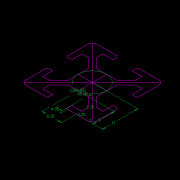
# Autodesk Inventor part: base2
Saved by Autodesk Inventor 2018 (Build 220112000, 112)
## iProperties
Created: 2022-02-17
Part Number: base2
Material: Generic
Document SubType Name: Modeling
Designer: kumpu
Density: 1 g/cm^3
Appearance: Default
Author: kumpu
Autodesk Inventor part; units mm, degrees
ref_plane "YZ Plane" through (0, 0, 0) normal (1, 0, 0) x (0, 1, 0)
ref_plane "XZ Plane" through (0, 0, 0) normal (0, 1, 0) x (-1, 0, 0)
ref_plane "XY Plane" through (0, 0, 0) normal (0, 0, 1) x (1, 0, 0)
sketch "Sketch1" plane through (0, 0, 0) normal (0, 1, 0) x (-1, 0, 0)
  line L0 (0, 0) -> (-14.4142, 14.4142)
  arc A0 (-13, 15) -> (-14.4142, 14.4142) centre (-13, 13) ccw
  line L1 (-13, 15) -> (-4.55, 15)
  line L2 (-4.55, 15) -> (-4, 14.45)
  line L3 (-4, 14.45) -> (-4, 12.75)
  line L4 (-4, 12.75) -> (-8.25, 12.75)
  line L5 (-8.25, 12.75) -> (-8.25, 10.0178)
  line L6 (-8.25, 10.0178) -> (-4.2322, 6)
  line L7 (-4.2322, 6) -> (0, 6)
  line L8 (0, 6) -> (0, 0)
  line L9 (0, 0) -> (14.4142, 14.4142)
  arc A1 (14.4142, 14.4142) -> (13, 15) centre (13, 13) ccw
  line L10 (13, 15) -> (4.55, 15)
  line L11 (4.55, 15) -> (4, 14.45)
  line L12 (4, 14.45) -> (4, 12.75)
  line L13 (4, 12.75) -> (8.25, 12.75)
  line L14 (8.25, 12.75) -> (8.25, 10.0178)
  line L15 (8.25, 10.0178) -> (4.2322, 6)
  line L16 (4.2322, 6) -> (0, 6)
  line L17 (-14.45, 4) -> (-12.75, 4)
  line L18 (-15, 4.55) -> (-14.45, 4)
  line L19 (-6, 4.2322) -> (-6, 0)
  line L20 (-6, 0) -> (0, 0)
  line L21 (-12.75, 4) -> (-12.75, 8.25)
  line L22 (-12.75, 8.25) -> (-10.0178, 8.25)
  line L23 (-10.0178, 8.25) -> (-6, 4.2322)
  line L24 (-15, 13) -> (-15, 4.55)
  arc A2 (-14.4142, 14.4142) -> (-15, 13) centre (-13, 13) ccw
  line L25 (0, 0) -> (-14.4142, 14.4142)
  line L26 (0, 0) -> (-14.4142, -14.4142)
  arc A3 (-15, -13) -> (-14.4142, -14.4142) centre (-13, -13) ccw
  line L27 (-6, -4.2322) -> (-6, 0)
  line L28 (-14.45, -4) -> (-12.75, -4)
  line L29 (-15, -4.55) -> (-14.45, -4)
  line L30 (-10.0178, -8.25) -> (-6, -4.2322)
  line L31 (-12.75, -8.25) -> (-10.0178, -8.25)
  line L32 (-12.75, -4) -> (-12.75, -8.25)
  line L33 (-15, -13) -> (-15, -4.55)
  line L34 (-4, -14.45) -> (-4, -12.75)
  line L35 (-4.55, -15) -> (-4, -14.45)
  line L36 (-4.2322, -6) -> (0, -6)
  line L37 (0, -6) -> (0, 0)
  line L38 (-4, -12.75) -> (-8.25, -12.75)
  line L39 (-8.25, -12.75) -> (-8.25, -10.0178)
  line L40 (-8.25, -10.0178) -> (-4.2322, -6)
  line L41 (-13, -15) -> (-4.55, -15)
  arc A4 (-14.4142, -14.4142) -> (-13, -15) centre (-13, -13) ccw
  line L42 (0, 0) -> (-14.4142, -14.4142)
  line L43 (0, 0) -> (14.4142, -14.4142)
  arc A5 (13, -15) -> (14.4142, -14.4142) centre (13, -13) ccw
  line L44 (4.2322, -6) -> (0, -6)
  line L45 (4, -14.45) -> (4, -12.75)
  line L46 (4.55, -15) -> (4, -14.45)
  line L47 (8.25, -10.0178) -> (4.2322, -6)
  line L48 (8.25, -12.75) -> (8.25, -10.0178)
  line L49 (4, -12.75) -> (8.25, -12.75)
  line L50 (13, -15) -> (4.55, -15)
  line L51 (14.45, -4) -> (12.75, -4)
  line L52 (15, -4.55) -> (14.45, -4)
  line L53 (6, -4.2322) -> (6, 0)
  line L54 (6, 0) -> (0, 0)
  line L55 (12.75, -4) -> (12.75, -8.25)
  line L56 (12.75, -8.25) -> (10.0178, -8.25)
  line L57 (10.0178, -8.25) -> (6, -4.2322)
  line L58 (15, -13) -> (15, -4.55)
  arc A6 (14.4142, -14.4142) -> (15, -13) centre (13, -13) ccw
  line L59 (0, 0) -> (14.4142, -14.4142)
  line L60 (0, 0) -> (14.4142, 14.4142)
  arc A7 (15, 13) -> (14.4142, 14.4142) centre (13, 13) ccw
  line L61 (6, 4.2322) -> (6, 0)
  line L62 (14.45, 4) -> (12.75, 4)
  line L63 (15, 4.55) -> (14.45, 4)
  line L64 (10.0178, 8.25) -> (6, 4.2322)
  line L65 (12.75, 8.25) -> (10.0178, 8.25)
  line L66 (12.75, 4) -> (12.75, 8.25)
  line L67 (15, 13) -> (15, 4.55)
  dimension "d0" = 45
  dimension "d1" = 1.25
  dimension "d2" = 2
  dimension "d4" = 9
  dimension "d5" = 15
  dimension "d6" = 4.55
  dimension "d7" = 4
  dimension "d8" = 8.25
  dimension "d9" = 2.25
  dimension "d12" = 360
  constraints: 136 end point, 16 point on circle, 9 symmetric about line, 8 centre point, 8 point on line, 4 perpendicular, 2 coincident, 2 parallel, 1 horizontal, 1 tangent, 1 vertical, 156 other
  measures "d0" angle of L0 L8
  measures "d1" distance between parallel lines of L0 L6
  measures "d2" radius of A0
  measures "d4" distance between parallel lines of L1 L7
  measures "d5" distance from line of L0.start L1
  measures "d6" distance from line of L8 L1.end
  measures "d7" distance between parallel lines of L8 L3
  measures "d8" distance between parallel lines of L8 L5
  measures "d9" distance between parallel lines of L1 L4
extrude "Extrusion1" add sketch "Sketch1" along normal blind 245.9
body "Solid1"
